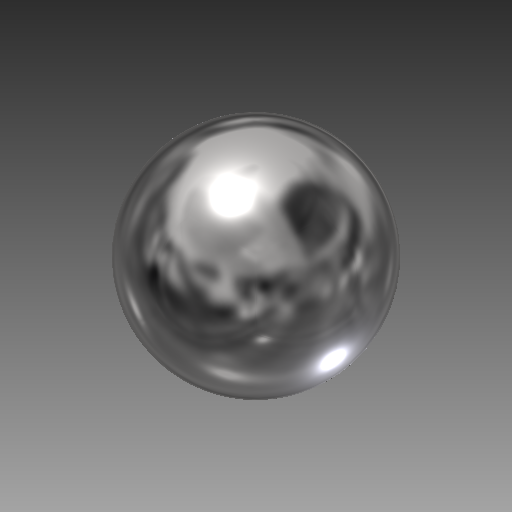
# Autodesk Inventor part: MF85ZZ Ball
Saved by Autodesk Inventor 2018 (Build 220112000, 112)
## iProperties
Category: PARTsolutions
Company: NSK_RB
Created: 2016-04-26
Part Number: MF85ZZ Ball
Catalog Web Link: www.cadenas.de
Description: shielded_type_zz_zzs_B-
Vendor: NSK_RB
Document SubType Name: Modeling
Designer: psAdmin
Manufacturer: NSK_RB
Mass: 0.0029582 g
Surface Area: 0.0254469 cm^2
Volume: 0.000381704 cm^3
Density: 7.75 g/cm^3
Material: ステンレス鋼 440C
Appearance: 半つや出し
PSOL_IDENT_0: {$CADENAS_DATA\23d-libs\nsk_rb\roller_bearings\deep_groove_bb\exstra_small_miniatur_bb\metric_design
PSOL_IDENT_1: _with_flange\shielded_type_zz_zzs_b_1.prj},181 {VTYP=3D},{NB=MF85ZZ Ball},{LINA=MF85ZZ Ball},{NN=shi
PSOL_IDENT_2: elded_type_zz_zzs_B},{DATE=18.06.2013 02:54:38},{GEOMDATE=04.01.2008 00:00:00},{VERSION=},{LINEID=21
PSOL_IDENT_3: 0},{LINESUBID=-1},{WBVAR=}  {NB=MF85ZZ Ball},{LINA=MF85ZZ Ball},{KT=DUMMY},{IDNR=},{STAN=},{ORDER=MF
PSOL_IDENT_4: 85ZZ},{SD=5.0},{X=5.0},{D=8},{DD=8},{DD1=0.0},{D2=9.2},{DD2=9.2},{B=0.0},{B1=2.5},{CC1=0.0},{C2=0.6}
PSOL_IDENT_5: ,{CC2=0.6},{R=0.00},{R1=0.10},{DI1=5.80},{DI2=5.80},{SDE1=7.00},{SDE2=7.40},{CR1=310},{COR1=120},{CR
PSOL_IDENT_6: 2=31},{COR2=12.0},{LG=53000},{LO=63000},{DA=0.0},{DB=5.8},{RA=0.00},{RB=0.10},{MASS=0.41},{SC=1}
NN: shielded_type_zz_zzs_B
NB: MF85ZZ Ball
NBSYN: $ORDER. Ball
LINA: MF85ZZ Ball
ORDER: MF85ZZ
SD: 5.0
X: 5.0
D: 8
DD: 8
DD1: 0.0
D2: 9.2
DD2: 9.2
B: 0.0
B1: 2.5
CC1: 0.0
C2: 0.6
CC2: 0.6
R: 0.00
R1: 0.10
DI1: 5.80
DI2: 5.80
SDE1: 7.00
SDE2: 7.40
CR1: 310
COR1: 120
CR2: 31
COR2: 12.0
LG: 53000
LO: 63000
DA: 0.0
DB: 5.8
RA: 0.00
RB: 0.10
MASS: 0.41
SC: 1
SUPPLIER: NSK_RB
ARTICLENO: MF85ZZ Ball
BOMINFO: MF85ZZ Ball
CREATOR: CADENAS GmbH
Title: MF85ZZ Ball
Author: Cadenas PARTsolutions
Autodesk Inventor part; units mm, degrees
sketch "Sketch_1" plane through (0, 0, 0) normal (0, 0, 1) x (1, 0, 0)
  line L0 (0.45, 0) -> (-0.45, 0)
  arc A0 (0.45, 0) -> (-0.45, 0) centre (0, 0) ccw
  line L1 (0.45, 0) -> (-0.45, 0)
  constraints: 4 end point, 2 point on circle, 1 centre point
revolve "Revolution1" add sketch "Sketch_1" angle 360 about axis through (0.45, 0, 0) along (1, 0, 0)
ref_plane "ip_st_1_XY" through (0, 0, 0) normal (-1, 0, 0) x (0, 0, -1)
ref_plane "ip_st_1_YZ" through (0, 0, 0) normal (0, 0, -1) x (0, -1, 0)
ref_plane "ip_st_1_ZX" through (0, 0, 0) normal (0, -1, 0) x (-1, 0, 0)
body "Solid1"
